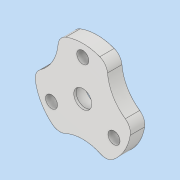
# Autodesk Inventor part: spoolPinionBearingHolder
Saved by Autodesk Inventor 2017 (Build 210142000, 142)
## iProperties
Created: 2016-11-06
Part Number: spoolPinionBearingHolder
Material: ABS Plastic
Document SubType Name: Modeling
Designer: techn
Density: 1.06 g/cm^3
Appearance: Smooth - White
Author: techn
Autodesk Inventor part; units mm, degrees
ref_plane "YZ Plane" through (0, 0, 0) normal (1, 0, 0) x (0, 1, 0)
ref_plane "XZ Plane" through (0, 0, 0) normal (0, 1, 0) x (-1, 0, 0)
ref_plane "XY Plane" through (0, 0, 0) normal (0, 0, 1) x (1, 0, 0)
sketch "Sketch1" plane through (0, 0, 0) normal (0, 0, 1) x (1, 0, 0)
  circle A0 centre (0, 0) radius 3.302
  line L0 (0, 0) -> (0, 9.525)
  circle A1 centre (0, 9.525) radius 1.5875
  circle A2 centre (-8.2489, -4.7625) radius 1.5875
  circle A3 centre (8.2489, -4.7625) radius 1.5875
  circle A4 centre (0, 0) radius 12.7
  dimension "d0" = 6.604
  dimension "d1" = 9.525
  dimension "d2" = 3.175
  dimension "d5" = 360
  dimension "d7" = 25.4
  constraints: 5 centre point, 3 coincident, 2 end point, 1 vertical, 7 other
  measures "d0" diameter of A0
  measures "d1" distance of L0.start L0.end
  measures "d2" diameter of A1
  measures "d7" diameter of A4
extrude "Extrusion1" add sketch "Sketch1" along normal blind 3.175
sketch "Sketch2" plane through (0, 0, 3.175) normal (0, 0, 1) x (1, 0, 0)
  circle A0 centre (0, 0) radius 3.302 projected
  circle A1 centre (8.2489, -4.7625) radius 1.5875 projected
  circle A2 centre (-8.2489, -4.7625) radius 1.5875 projected
  circle A3 centre (0, 9.525) radius 1.5875 projected
  circle A4 centre (0, 0) radius 12.7 projected
  circle A5 centre (0, 0) radius 2.3813
  dimension "d10" = 4.7625
  constraints: 1 centre point, 1 coincident
  measures "d10" diameter of A5
extrude "Extrusion2" add sketch "Sketch2" along normal blind 0.635 contours A0 | A4
chamfer "Chamfer1" distance 1.27 angle 45 3 edges at (-1.5875, 9.525, 0) (-9.8364, -4.7625, 0) (6.6614, -4.7625, 0)
sketch "Sketch3" plane through (0, 0, 0) normal (0, 0, -1) x (-1, 0, 0)
  line L0 (0, 0) -> (17.5976, 10.16)
  line L1 (0, 0) -> (20.32, 0) construction
  circle A0 centre (17.5976, 10.16) radius 11.1125
  circle A1 centre (-17.5976, 10.16) radius 11.1125
  circle A2 centre (0, -20.32) radius 11.1125
  dimension "d16" = 20.32
  dimension "d17" = 30
  dimension "d18" = 22.225
  dimension "d21" = 360
  constraints: 4 end point, 3 centre point, 1 coincident, 1 equal length, 1 horizontal, 7 other
  measures "d16" distance of L0.start L0.end
  measures "d17" angle of L1 L0
  measures "d18" diameter of A0
extrude "Extrusion3" cut sketch "Sketch3" against normal blind 25.4
fillet "Fillet1" radius 3.175 6 edges at (-12.6986, 0.1857, 1.905) (-6.5101, 10.9045, 1.905) (12.6986, 0.1857, 1.905) (6.5101, 10.9045, 1.905) (6.1885, -11.0902, 1.905) (-6.1885, -11.0902, 1.905)
body "Solid1"
